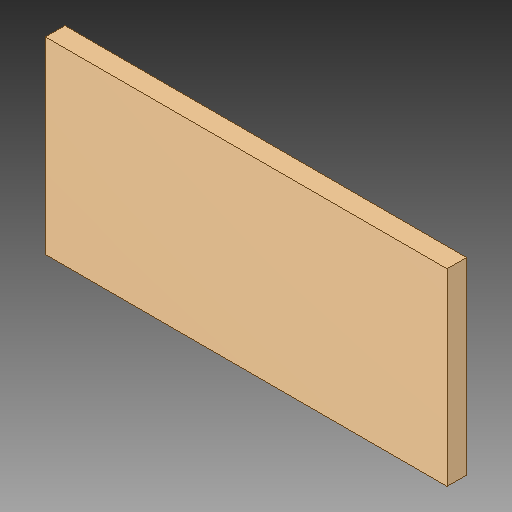
# Autodesk Inventor part: LMD18200T
Saved by Autodesk Inventor 2017 (Build 210142000, 142)
## iProperties
Created: 2019-06-13
Part Number: LMD18200T
Material: Generic
Document SubType Name: Modeling
Designer: Marc
Density: 1 g/cm^3
Appearance: TO-220-11, LMD18200T
Author: Marc
Autodesk Inventor part; units mm, degrees
ref_plane "YZ Plane" through (0, 0, 0) normal (1, 0, 0) x (0, 1, 0)
ref_plane "XZ Plane" through (0, 0, 0) normal (0, 1, 0) x (-1, 0, 0)
ref_plane "XY Plane" through (0, 0, 0) normal (0, 0, 1) x (1, 0, 0)
sketch "TO-220-11, LMD18200T_54" plane through (0, 0, 0) normal (0, 0, 1) x (1, 0, 0)
  line L0 (-9.8615, 6.8072) -> (10.7125, 6.8072)
  line L1 (10.7125, 6.8072) -> (10.7125, -2.8448)
  line L2 (10.7125, -2.8448) -> (-9.8615, -2.8448)
  line L3 (-9.8615, -2.8448) -> (-9.8615, 6.8072)
  constraints: 8 end point
extrude "Extrusion1" add sketch "TO-220-11, LMD18200T_54" along normal blind 1
body "Solid1"
